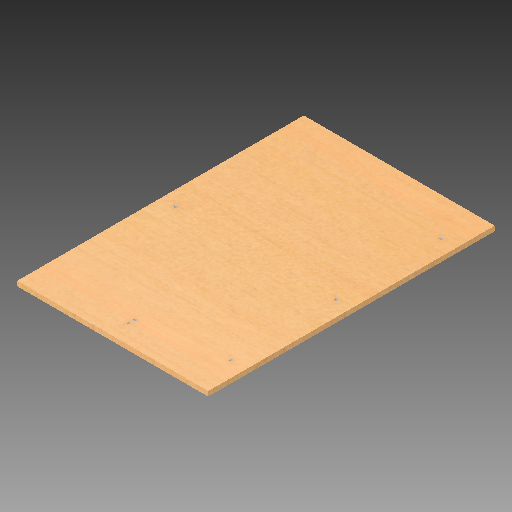
# Autodesk Inventor part: toit
Saved by Autodesk Inventor 2017 (Build 210142000, 142)
## iProperties
Created: 2018-04-02
Part Number: toit
Material: Generic
Document SubType Name: Modeling
Designer: franc
Density: 1 g/cm^3
Appearance: Default
Author: franc
Autodesk Inventor part; units mm, degrees
ref_plane "YZ Plane" through (0, 0, 0) normal (1, 0, 0) x (0, 1, 0)
ref_plane "XZ Plane" through (0, 0, 0) normal (0, 1, 0) x (-1, 0, 0)
ref_plane "XY Plane" through (0, 0, 0) normal (0, 0, 1) x (1, 0, 0)
sketch "Esquisse1" plane through (0, 0, 0) normal (0, 1, 0) x (-1, 0, 0)
  line L0 (110.1985, 107.2202) -> (-89.8015, 107.2202)
  line L1 (-89.8015, 107.2202) -> (-89.8015, -192.7798)
  line L2 (-89.8015, -192.7798) -> (110.1985, -192.7798)
  line L3 (110.1985, -192.7798) -> (110.1985, 107.2202)
  point P0 (0, 0)
  dimension "d0" = 300
  dimension "d1" = 200
  constraints: 8 end point, 2 parallel, 1 horizontal, 1 perpendicular
  measures "d0" distance of L2.end L0.start
  measures "d1" distance of L0.start L0.end
extrude "Extrusion1" add sketch "Esquisse1" along normal blind 5
sketch "Esquisse2" plane through (0, 0, 0) normal (0, -1, 0) x (1, 0, 0)
  circle A0 centre (-94.1985, -42.7798) radius 1.5
  circle A1 centre (73.8015, -42.7798) radius 1.5
  circle A2 centre (73.8015, 67.2202) radius 1.5
  circle A3 centre (73.8015, -152.7798) radius 1.5
  line L0 (-110.1985, -192.7798) -> (-110.1985, 107.2202) projected
  line L1 (89.8015, -192.7798) -> (-110.1985, -192.7798) projected
  line L2 (89.8015, 107.2202) -> (89.8015, -192.7798) projected
  line L3 (-110.1985, 107.2202) -> (89.8015, 107.2202) projected
  point P0 (0, 0)
  dimension "d4" = 16
  dimension "d5" = 150
  dimension "d6" = 16
  dimension "d7" = 16
  dimension "d8" = 16
  dimension "d9" = 40
  dimension "d10" = 150
  dimension "d11" = 40
  constraints: 4 centre point
  measures "d4" distance from line of L0 A0.centre
  measures "d5" distance from line of L1 A0.centre
  measures "d6" distance from line of L2 A2.centre
  measures "d7" distance from line of L2 A1.centre
  measures "d8" distance from line of L2 A3.centre
  measures "d9" distance from line of L1 A3.centre
  measures "d10" distance from line of L1 A1.centre
  measures "d11" distance from line of L3 A2.centre
extrude "Extrusion2" cut sketch "Esquisse2" against normal through all contours A0 | A1 | A2 | A3
sketch "Sketch4" plane through (0, 5, 0) normal (0, 1, 0) x (1, 0, 0)
  circle A0 centre (-13.1985, -87.2202) radius 1.5001 projected
  circle A1 centre (-13.1985, -80.7202) radius 1.5 projected
  point P0 (0, 0)
extrude "Extrusion4" cut sketch "Sketch4" against normal through all
